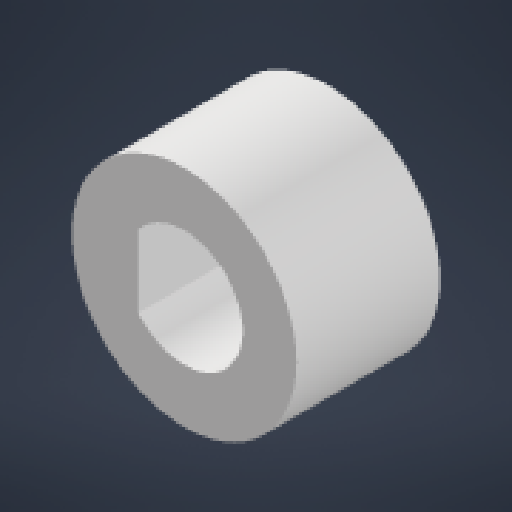
# Autodesk Inventor part: Pladeholder
Saved by Autodesk Inventor 2026.1 (Build 301233020, 233B)
## iProperties
Created: 2025-12-03
Part Number: Pladeholder
Material: Generic
Document SubType Name: Modeling
Designer: Mikke
Density: 1 g/cm^3
Appearance: Default
Author: Mikke
Autodesk Inventor part; units mm, degrees
ref_plane "YZ Plane" through (0, 0, 0) normal (1, 0, 0) x (0, 1, 0)
ref_plane "XZ Plane" through (0, 0, 0) normal (0, 1, 0) x (-1, 0, 0)
ref_plane "XY Plane" through (0, 0, 0) normal (0, 0, 1) x (1, 0, 0)
sketch "Sketch1" plane through (0, 0, 0) normal (0, 0, 1) x (1, 0, 0)
  arc A0 (-2.55, -2.0149) -> (-2.55, 2.0149) centre (0, 0) ccw projected
  line L0 (-2.55, 2.0149) -> (-2.55, -2.0149) projected
  arc A1 (-9.55, -3.7229) -> (-9.55, 3.7229) centre (0, 0) ccw
  line L1 (-9.55, -3.7229) -> (-9.55, 3.7229)
  point P0 (0, 0)
  dimension "d4" = 7
  constraints: 2 end point, 2 point on circle, 1 centre point, 1 other
  measures "d4" radial gap between concentric circles of A0 A1
extrude "Extrusion1" add sketch "Sketch1" along normal blind 12
sketch "Sketch2" plane through (-9.55, -3.7229, 0) normal (-1, 0, 0) x (0, 0, 1)
  line L0 (0, 7.4458) -> (0, 0) projected
  line L1 (0, 0) -> (12, 0) projected
  line L2 (12, 7.4458) -> (12, 0) projected
  line L3 (0, 7.4458) -> (12, 7.4458) projected
  circle A0 centre (6, 3.7229) radius 3.25
  point P0 (0, 3.7229)
  constraints: 1 centre point
extrude "Extrusion2" cut sketch "Sketch2" against normal blind 10.4125 contours A0
sketch "Sketch3" plane through (0, 0, 12) normal (0, 0, 1) x (1, 0, 0)
  arc A0 (-2.55, -2.0149) -> (-2.55, 2.0149) centre (0, 0) ccw projected
  line L0 (-2.55, 2.0149) -> (-2.55, -2.0149) projected
  line L1 (-9.55, 3.7229) -> (-9.55, -3.7229) projected
  arc A1 (-9.55, -3.7229) -> (-9.55, 3.7229) centre (0, 0) ccw projected
  line L2 (-2.55, -2.0149) -> (-2.55, 2.0149) projected
  arc A2 (-2.55, -2.0149) -> (-2.55, 2.0149) centre (0, 0) ccw projected
  line L3 (0, 10.25) -> (0, 3.25)
  circle A3 centre (0, 6.75) radius 2
  circle A4 centre (6.75, 0) radius 2
  circle A5 centre (0, -6.75) radius 2
  point P0 (0, 0)
  dimension "d7" = 4
  dimension "d10" = 180
  constraints: 3 centre point, 2 end point, 2 point on circle, 1 midpoint, 1 vertical, 5 other
  measures "d7" diameter of A3
extrude "Extrusion3" cut sketch "Sketch3" against normal blind 5.7 contours A3 L3 | L3 A3 | A4 | A5
body "Solid1"
